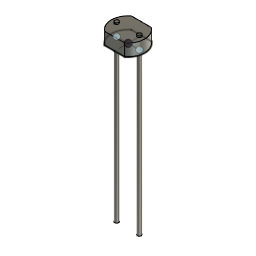
2020_09_21_LightResistor v3 (Autodesk Fusion 360 design; units mm, degrees)
Autodesk Fusion 360 part; units mm, degrees
sketch "LightResistorMeasurement" plane through (0, 0, 0) normal (0, 0, 1) x (1, 0, 0)
  line L0 (0, 0) -> (0.0874, 0)
  line L1 (0, 0) -> (0, 2) construction
  line L2 (0, 0) -> (0, -2) construction
  line L3 (0, 2) -> (1.5, 2)
  line L4 (0, 2) -> (-1.5, 2)
  line L5 (0, -2) -> (1.5, -2)
  line L6 (0, -2) -> (-1.5, -2)
  arc A0 (-1.5, 2) -> (-1.5, -2) centre (0, 0) ccw
  arc A1 (1.5, -2) -> (1.5, 2) centre (0, 0) ccw
  line L7 (0, 0) -> (2, 0) construction
  line L8 (0, 0) -> (-2, 0) construction
  circle A2 centre (-1.7, 0) radius 0.3
  circle A3 centre (1.7, 0) radius 0.3
  dimension "d1" = 5
  dimension "d2" = 2
  dimension "d3" = 2
  dimension "d4" = 2
  dimension "d5" = 0.6
  dimension "d6" = 0.6
  constraint coincident L0.start L1.start
  constraint horizontal L0
  constraint perpendicular L0 L1
  constraint perpendicular L0 L2
  constraint equal L1 L2
  constraint perpendicular L1 L3
  constraint perpendicular L1 L4
  constraint coincident L5.end A0
  constraint perpendicular L2 L5
  constraint perpendicular L2 L6
  constraint concentric A0 A1
  constraint perpendicular L1 L7
  constraint perpendicular L2 L8
  constraint coincident L8.end A2
  constraint coincident L7.end A3
  measures "d1" diameter of A0
  measures "d2" distance of L0.start L1.end
  measures "d3" distance of L0.start L7.end
  measures "d4" distance of L0.start L8.end
  measures "d5" diameter of A2
  measures "d6" diameter of A3
extrude "Extrude1" add sketch "LightResistorMeasurement" along normal blind 1.8 contours L3 L4 L5 L6 A0 A1 | A2 | A3
extrude "Extrude2" add sketch "LightResistorMeasurement" against normal blind 24 contours A2 | A3
extrude "Extrude3" add sketch "LightResistorMeasurement" along normal blind 2 contours A2 | A3
named bodies: "LightResistor"
